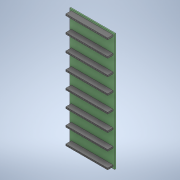
# Autodesk Inventor part: DaughterBoard
Saved by Autodesk Inventor 2020 (Build 240168000, 168)
## iProperties
Created: 2019-12-15
Part Number: DaughterBoard
Material: Generic
Document SubType Name: Modeling
Designer: torto
Density: 1 g/cm^3
Appearance: Default
Author: torto
Autodesk Inventor part; units mm, degrees
ref_plane "YZ Plane" through (0, 0, 0) normal (1, 0, 0) x (0, 1, 0)
ref_plane "XZ Plane" through (0, 0, 0) normal (0, 1, 0) x (-1, 0, 0)
ref_plane "XY Plane" through (0, 0, 0) normal (0, 0, 1) x (1, 0, 0)
sketch "General PCB Dimensions" plane through (0, 0, 0) normal (0, 0, 1) x (1, 0, 0)
  line L0 (0, 0) -> (71.12, 0)
  line L1 (71.12, 0) -> (71.12, 185.42)
  line L2 (71.12, 185.42) -> (0, 185.42)
  line L3 (0, 185.42) -> (0, 0)
  line L4 (71.12, 185.42) -> (50.8, 185.42) construction
  line L5 (71.12, 181.61) -> (71.12, 185.42) construction
  dimension "PcbLength" = 71.12
  dimension "PcbHeight" = 185.42
  constraints: 12 end point, 2 horizontal, 2 parallel, 1 perpendicular
  measures "PcbLength" distance of L1.end L2.end
  measures "PcbHeight" distance of L0.end L1.end
extrude "PCB" add sketch "General PCB Dimensions" along normal blind 1.6
sketch "Female Headers" plane through (0, 0, 1.6) normal (0, 0, 1) x (1, 0, 0)
  line L0 (0, 0) -> (71.12, 0)
  line L1 (71.12, 0) -> (71.12, 185.42)
  line L2 (71.12, 185.42) -> (0, 185.42)
  line L3 (0, 185.42) -> (0, 0)
  line L4 (71.12, 185.42) -> (35.56, 185.42) construction
  line L5 (35.56, 185.42) -> (35.56, 181.61) construction
  line L6 (35.56, 181.61) -> (71.12, 181.61) construction
  line L7 (71.12, 181.61) -> (71.12, 185.42) construction
  line L8 (2.54, 182.88) -> (68.58, 182.88)
  line L9 (68.58, 182.88) -> (68.58, 180.34)
  line L10 (68.58, 180.34) -> (2.54, 180.34)
  line L11 (2.54, 180.34) -> (2.54, 182.88)
  line L12 (2.54, 182.88) -> (68.58, 180.34) construction
  line L13 (68.58, 182.88) -> (2.54, 180.34) construction
  line L14 (68.58, 182.88) -> (66.04, 182.88)
  line L15 (66.04, 182.88) -> (66.04, 180.34)
  line L16 (66.04, 180.34) -> (68.58, 180.34)
  line L17 (68.58, 180.34) -> (68.58, 182.88)
  line L18 (67.31, 182.88) -> (67.31, 180.34) construction
  line L19 (66.9925, 181.9275) -> (67.6275, 181.9275)
  line L20 (67.6275, 181.9275) -> (67.6275, 181.2925)
  line L21 (67.6275, 181.2925) -> (66.9925, 181.2925)
  line L22 (66.9925, 181.2925) -> (66.9925, 181.9275)
  line L23 (66.9925, 181.9275) -> (67.6275, 181.2925) construction
  line L24 (67.6275, 181.9275) -> (66.9925, 181.2925) construction
  line L25 (63.5, 182.88) -> (63.5, 180.34)
  line L26 (66.04, 182.88) -> (66.04, 180.34)
  line L27 (64.4525, 181.2925) -> (64.4525, 181.9275)
  line L28 (64.4525, 181.9275) -> (65.0875, 181.9275)
  line L29 (65.0875, 181.9275) -> (65.0875, 181.2925)
  line L30 (65.0875, 181.2925) -> (64.4525, 181.2925)
  line L31 (60.96, 182.88) -> (60.96, 180.34)
  line L32 (63.5, 182.88) -> (63.5, 180.34)
  line L33 (61.9125, 181.2925) -> (61.9125, 181.9275)
  line L34 (61.9125, 181.9275) -> (62.5475, 181.9275)
  line L35 (62.5475, 181.9275) -> (62.5475, 181.2925)
  line L36 (62.5475, 181.2925) -> (61.9125, 181.2925)
  line L37 (58.42, 182.88) -> (58.42, 180.34)
  line L38 (60.96, 182.88) -> (60.96, 180.34)
  line L39 (59.3725, 181.2925) -> (59.3725, 181.9275)
  line L40 (59.3725, 181.9275) -> (60.0075, 181.9275)
  line L41 (60.0075, 181.9275) -> (60.0075, 181.2925)
  line L42 (60.0075, 181.2925) -> (59.3725, 181.2925)
  line L43 (55.88, 182.88) -> (55.88, 180.34)
  line L44 (58.42, 182.88) -> (58.42, 180.34)
  line L45 (56.8325, 181.2925) -> (56.8325, 181.9275)
  line L46 (56.8325, 181.9275) -> (57.4675, 181.9275)
  line L47 (57.4675, 181.9275) -> (57.4675, 181.2925)
  line L48 (57.4675, 181.2925) -> (56.8325, 181.2925)
  line L49 (53.34, 182.88) -> (53.34, 180.34)
  line L50 (55.88, 182.88) -> (55.88, 180.34)
  line L51 (54.2925, 181.2925) -> (54.2925, 181.9275)
  line L52 (54.2925, 181.9275) -> (54.9275, 181.9275)
  line L53 (54.9275, 181.9275) -> (54.9275, 181.2925)
  line L54 (54.9275, 181.2925) -> (54.2925, 181.2925)
  line L55 (50.8, 182.88) -> (50.8, 180.34)
  line L56 (53.34, 182.88) -> (53.34, 180.34)
  line L57 (51.7525, 181.2925) -> (51.7525, 181.9275)
  line L58 (51.7525, 181.9275) -> (52.3875, 181.9275)
  line L59 (52.3875, 181.9275) -> (52.3875, 181.2925)
  line L60 (52.3875, 181.2925) -> (51.7525, 181.2925)
  line L61 (48.26, 182.88) -> (48.26, 180.34)
  line L62 (50.8, 182.88) -> (50.8, 180.34)
  line L63 (49.2125, 181.2925) -> (49.2125, 181.9275)
  line L64 (49.2125, 181.9275) -> (49.8475, 181.9275)
  line L65 (49.8475, 181.9275) -> (49.8475, 181.2925)
  line L66 (49.8475, 181.2925) -> (49.2125, 181.2925)
  line L67 (45.72, 182.88) -> (45.72, 180.34)
  line L68 (48.26, 182.88) -> (48.26, 180.34)
  line L69 (46.6725, 181.2925) -> (46.6725, 181.9275)
  line L70 (46.6725, 181.9275) -> (47.3075, 181.9275)
  line L71 (47.3075, 181.9275) -> (47.3075, 181.2925)
  line L72 (47.3075, 181.2925) -> (46.6725, 181.2925)
  line L73 (43.18, 182.88) -> (43.18, 180.34)
  line L74 (45.72, 182.88) -> (45.72, 180.34)
  line L75 (44.1325, 181.2925) -> (44.1325, 181.9275)
  line L76 (44.1325, 181.9275) -> (44.7675, 181.9275)
  line L77 (44.7675, 181.9275) -> (44.7675, 181.2925)
  line L78 (44.7675, 181.2925) -> (44.1325, 181.2925)
  line L79 (40.64, 182.88) -> (40.64, 180.34)
  line L80 (43.18, 182.88) -> (43.18, 180.34)
  line L81 (41.5925, 181.2925) -> (41.5925, 181.9275)
  line L82 (41.5925, 181.9275) -> (42.2275, 181.9275)
  line L83 (42.2275, 181.9275) -> (42.2275, 181.2925)
  line L84 (42.2275, 181.2925) -> (41.5925, 181.2925)
  line L85 (38.1, 182.88) -> (38.1, 180.34)
  line L86 (40.64, 182.88) -> (40.64, 180.34)
  line L87 (39.0525, 181.2925) -> (39.0525, 181.9275)
  line L88 (39.0525, 181.9275) -> (39.6875, 181.9275)
  line L89 (39.6875, 181.9275) -> (39.6875, 181.2925)
  line L90 (39.6875, 181.2925) -> (39.0525, 181.2925)
  line L91 (35.56, 182.88) -> (35.56, 180.34)
  line L92 (38.1, 182.88) -> (38.1, 180.34)
  line L93 (36.5125, 181.2925) -> (36.5125, 181.9275)
  line L94 (36.5125, 181.9275) -> (37.1475, 181.9275)
  line L95 (37.1475, 181.9275) -> (37.1475, 181.2925)
  line L96 (37.1475, 181.2925) -> (36.5125, 181.2925)
  line L97 (33.02, 182.88) -> (33.02, 180.34)
  line L98 (35.56, 182.88) -> (35.56, 180.34)
  line L99 (33.9725, 181.2925) -> (33.9725, 181.9275)
  line L100 (33.9725, 181.9275) -> (34.6075, 181.9275)
  line L101 (34.6075, 181.9275) -> (34.6075, 181.2925)
  line L102 (34.6075, 181.2925) -> (33.9725, 181.2925)
  line L103 (30.48, 182.88) -> (30.48, 180.34)
  line L104 (33.02, 182.88) -> (33.02, 180.34)
  line L105 (31.4325, 181.2925) -> (31.4325, 181.9275)
  line L106 (31.4325, 181.9275) -> (32.0675, 181.9275)
  line L107 (32.0675, 181.9275) -> (32.0675, 181.2925)
  line L108 (32.0675, 181.2925) -> (31.4325, 181.2925)
  line L109 (27.94, 182.88) -> (27.94, 180.34)
  line L110 (30.48, 182.88) -> (30.48, 180.34)
  line L111 (28.8925, 181.2925) -> (28.8925, 181.9275)
  line L112 (28.8925, 181.9275) -> (29.5275, 181.9275)
  line L113 (29.5275, 181.9275) -> (29.5275, 181.2925)
  line L114 (29.5275, 181.2925) -> (28.8925, 181.2925)
  line L115 (25.4, 182.88) -> (25.4, 180.34)
  line L116 (27.94, 182.88) -> (27.94, 180.34)
  line L117 (26.3525, 181.2925) -> (26.3525, 181.9275)
  line L118 (26.3525, 181.9275) -> (26.9875, 181.9275)
  line L119 (26.9875, 181.9275) -> (26.9875, 181.2925)
  line L120 (26.9875, 181.2925) -> (26.3525, 181.2925)
  line L121 (22.86, 182.88) -> (22.86, 180.34)
  line L122 (25.4, 182.88) -> (25.4, 180.34)
  line L123 (23.8125, 181.2925) -> (23.8125, 181.9275)
  line L124 (23.8125, 181.9275) -> (24.4475, 181.9275)
  line L125 (24.4475, 181.9275) -> (24.4475, 181.2925)
  line L126 (24.4475, 181.2925) -> (23.8125, 181.2925)
  line L127 (20.32, 182.88) -> (20.32, 180.34)
  line L128 (22.86, 182.88) -> (22.86, 180.34)
  line L129 (21.2725, 181.2925) -> (21.2725, 181.9275)
  line L130 (21.2725, 181.9275) -> (21.9075, 181.9275)
  line L131 (21.9075, 181.9275) -> (21.9075, 181.2925)
  line L132 (21.9075, 181.2925) -> (21.2725, 181.2925)
  line L133 (17.78, 182.88) -> (17.78, 180.34)
  line L134 (20.32, 182.88) -> (20.32, 180.34)
  line L135 (18.7325, 181.2925) -> (18.7325, 181.9275)
  line L136 (18.7325, 181.9275) -> (19.3675, 181.9275)
  line L137 (19.3675, 181.9275) -> (19.3675, 181.2925)
  line L138 (19.3675, 181.2925) -> (18.7325, 181.2925)
  line L139 (15.24, 182.88) -> (15.24, 180.34)
  line L140 (17.78, 182.88) -> (17.78, 180.34)
  line L141 (16.1925, 181.2925) -> (16.1925, 181.9275)
  line L142 (16.1925, 181.9275) -> (16.8275, 181.9275)
  line L143 (16.8275, 181.9275) -> (16.8275, 181.2925)
  line L144 (16.8275, 181.2925) -> (16.1925, 181.2925)
  line L145 (12.7, 182.88) -> (12.7, 180.34)
  line L146 (15.24, 182.88) -> (15.24, 180.34)
  line L147 (13.6525, 181.2925) -> (13.6525, 181.9275)
  line L148 (13.6525, 181.9275) -> (14.2875, 181.9275)
  line L149 (14.2875, 181.9275) -> (14.2875, 181.2925)
  line L150 (14.2875, 181.2925) -> (13.6525, 181.2925)
  line L151 (10.16, 182.88) -> (10.16, 180.34)
  line L152 (12.7, 182.88) -> (12.7, 180.34)
  line L153 (11.1125, 181.2925) -> (11.1125, 181.9275)
  line L154 (11.1125, 181.9275) -> (11.7475, 181.9275)
  line L155 (11.7475, 181.9275) -> (11.7475, 181.2925)
  line L156 (11.7475, 181.2925) -> (11.1125, 181.2925)
  line L157 (7.62, 182.88) -> (7.62, 180.34)
  line L158 (10.16, 182.88) -> (10.16, 180.34)
  line L159 (8.5725, 181.2925) -> (8.5725, 181.9275)
  line L160 (8.5725, 181.9275) -> (9.2075, 181.9275)
  line L161 (9.2075, 181.9275) -> (9.2075, 181.2925)
  line L162 (9.2075, 181.2925) -> (8.5725, 181.2925)
  line L163 (5.08, 182.88) -> (5.08, 180.34)
  line L164 (7.62, 182.88) -> (7.62, 180.34)
  line L165 (6.0325, 181.2925) -> (6.0325, 181.9275)
  line L166 (6.0325, 181.9275) -> (6.6675, 181.9275)
  line L167 (6.6675, 181.9275) -> (6.6675, 181.2925)
  line L168 (6.6675, 181.2925) -> (6.0325, 181.2925)
  line L169 (2.54, 182.88) -> (2.54, 180.34)
  line L170 (5.08, 182.88) -> (5.08, 180.34)
  line L171 (3.4925, 181.2925) -> (3.4925, 181.9275)
  line L172 (3.4925, 181.9275) -> (4.1275, 181.9275)
  line L173 (4.1275, 181.9275) -> (4.1275, 181.2925)
  line L174 (4.1275, 181.2925) -> (3.4925, 181.2925)
  point P0 (67.31, 181.61)
  dimension "d26" = 71.12
  dimension "d27" = 185.42
  dimension "d28" = 35.56
  dimension "d29" = 3.81
  dimension "d30" = 66.04
  dimension "d31" = 2.54
  dimension "d32" = 2.54
  dimension "d33" = 2.54
  dimension "d34" = 0.635
  dimension "d35" = 0.635
  dimension "d36" = 2.54
  constraints: 350 end point, 10 parallel, 7 midpoint, 6 horizontal, 5 perpendicular, 1 coincident, 350 other
  measures "d26" distance of L1.end L2.end
  measures "d27" distance of L0.end L1.end
  measures "d28" distance of L6.end L5.end
  measures "d29" distance of L5.end L4.end
  measures "d30" distance of L9.end L10.end
  measures "d31" distance of L8.end L9.end
  measures "d32" distance of L16.end L15.end
  measures "d33" distance of L15.end L14.end
  measures "d34" distance of L20.end L21.end
  measures "d35" distance of L19.end L20.end
  measures "d36" distance of L14.end L25.start
extrude "Extrusion3" add sketch "Female Headers" along normal blind 8.636 contours L8 L163 L10 L11 | L8 L157 L10 L163 | L8 L151 L10 L157 | L8 L145 L10 L151 | L8 L139 L10 L145 | L8 L133 L10 L139 | L8 L127 L10 L133 | L8 L121 L10 L127 | L8 L115 L10 L121 | L8 L109 L10 L115 | L8 L103 L10 L109 | L8 L97 L10 L103 | L8 L91 L10 L97 | L8 L85 L10 L91 | L8 L79 L10 L85 | L8 L73 L10 L79 | L8 L67 L10 L73 | L8 L61 L10 L67 | L8 L55 L10 L61 | L8 L49 L10 L55 | L8 L43 L10 L49 | L8 L37 L10 L43 | L8 L31 L10 L37 | L8 L25 L10 L31 | L8 L15 L10 L25 | L8 L9 L10 L15
pattern_linear "Female Header Pattern" count 8 spacing 25.4 along (0, -1, 0) of "Extrusion3"
equation "\"d26\" = PcbLength"
equation "\"d27\" = PcbHeight"
equation "\"d28\" = 0.5 * d26"
equation "\"d32\" = d31"
equation "\"d33\" = d31"
equation "\"d35\" = d34"
equation "\"d36\" = d31"
body "Solid2"
